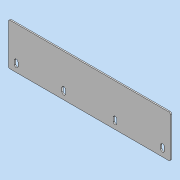
# Autodesk Inventor part: Scraper_Bar_Flat
Saved by Autodesk Inventor 2020 (Build 240168000, 168)
## iProperties
Created: 2021-06-14
Part Number: Scraper_Bar_Flat
Material: Generic
Document SubType Name: Modeling
Designer: magnarecta
Density: 1 g/cm^3
Appearance: Default
Author: magnarecta
Autodesk Inventor part; units mm, degrees
ref_plane "YZ Plane" through (0, 0, 0) normal (1, 0, 0) x (0, 1, 0)
ref_plane "XZ Plane" through (0, 0, 0) normal (0, 1, 0) x (-1, 0, 0)
ref_plane "XY Plane" through (0, 0, 0) normal (0, 0, 1) x (1, 0, 0)
sketch "スケッチ1" plane through (0, 0, 0) normal (0, 0, 1) x (1, 0, 0)
  line L0 (135.25, -40.8489) -> (135.25, -45.8489)
  arc A0 (130.75, -45.8489) -> (135.25, -45.8489) centre (133, -45.8489) ccw
  line L1 (130.75, -45.8489) -> (130.75, -40.8489)
  arc A1 (135.25, -40.8489) -> (130.75, -40.8489) centre (133, -40.8489) ccw
  line L2 (70.25, -40.8489) -> (70.25, -45.8489)
  arc A2 (65.75, -45.8489) -> (70.25, -45.8489) centre (68, -45.8489) ccw
  line L3 (65.75, -45.8489) -> (65.75, -40.8489)
  arc A3 (70.25, -40.8489) -> (65.75, -40.8489) centre (68, -40.8489) ccw
  line L4 (195.25, -40.8489) -> (195.25, -45.8489)
  arc A4 (190.75, -45.8489) -> (195.25, -45.8489) centre (193, -45.8489) ccw
  line L5 (190.75, -45.8489) -> (190.75, -40.8489)
  arc A5 (195.25, -40.8489) -> (190.75, -40.8489) centre (193, -40.8489) ccw
  line L6 (5.75, -45.8489) -> (5.75, -40.8489)
  arc A6 (10.25, -40.8489) -> (5.75, -40.8489) centre (8, -40.8489) ccw
  line L7 (10.25, -40.8489) -> (10.25, -45.8489)
  arc A7 (5.75, -45.8489) -> (10.25, -45.8489) centre (8, -45.8489) ccw
  arc A8 (203, -2) -> (201, 0) centre (201, -2) ccw
  line L8 (0, 0) -> (201, 0)
  arc A9 (0, 0) -> (-2, -2) centre (0, -2) ccw
  line L9 (-2, -51.3489) -> (-2, -2)
  arc A10 (-2, -51.3489) -> (0, -53.3489) centre (0, -51.3489) ccw
  line L10 (201, -53.3489) -> (0, -53.3489)
  arc A11 (201, -53.3489) -> (203, -51.3489) centre (201, -51.3489) ccw
  line L11 (203, -2) -> (203, -51.3489)
  constraints: 24 end point, 24 point on circle, 12 centre point
extrude "押し出し1" add sketch "スケッチ1" along normal blind 1.6
